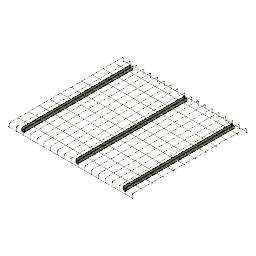
_Wire Rack.2c1b638f-f074-42f4-967c-a75b4d30ed14 (Autodesk Fusion 360 design; units mm, degrees)
Autodesk Fusion 360 part; units mm, degrees
note: some values were not read from the file. Set by a fixed rule: which sketch regions a step uses.
sketch "Sketch1" plane through (0, 0, 0) normal (1, 0, 0) x (0, 1, 0)
  circle A0 centre (0, 0) radius 2.5
  dimension "d1" = 5
  constraint coincident A0.centre origin
  measures "d1" diameter of A0
extrude "Extrude1" add sketch "Sketch1" against normal blind 1162.05 makes body 1
ref_plane "WorkPlane1" through (-4.5, 0, 0) normal (1, 0, 0) x (0, 1, 0)
sketch "Sketch2" plane through (-4.5, 0, 0) normal (1, 0, 0) x (0, 1, 0)
  circle A0 centre (0, 0) radius 2.5
  line L0 (0, 0) -> (2.5, 0)
  line L1 (5, -4.5) -> (5, 26.65)
  line L2 (11.35, 33) -> (1064.1038, 33)
  line L3 (1070.4538, 26.65) -> (1070.4538, -4.5)
  arc A1 (11.35, 33) -> (5, 26.65) centre (11.35, 26.65) ccw
  arc A2 (1070.4538, 26.65) -> (1064.1038, 33) centre (1064.1038, 26.65) ccw
  line L4 (5, -4.5) -> (-3, -4.5) construction
  point P0 (5, 33)
  point P1 (1070.4538, 33)
  dimension "d8" = 37.5
  dimension "d9" = 1065.4538
  dimension "d10" = 37.5
  dimension "d11" = 6.35
  dimension "d12" = 6.35
  constraint coincident A0.centre L0.start
  constraint coincident A0 L0.end
  constraint horizontal L0
  constraint perpendicular L1 L2
  constraint perpendicular L2 L3
  constraint coincident P0 L1
  constraint coincident P0 L2
  constraint tangent L1 A1
  constraint tangent L2 A1
  constraint coincident P1 L3
  constraint coincident P1 L2
  constraint tangent L3 A2
  constraint tangent L2 A2
  constraint perpendicular L1 L4
  measures "d8" distance of L1.start P0
  measures "d9" distance of P0 P1
  measures "d10" distance of P1 L3.end
  measures "d11" radius of A1
  measures "d12" radius of A2
ref_plane "WorkPlane2" through (-4.5, 1, -4.5) normal (0, 0, 1) x (0, -1, 0)
sketch "Sketch3" plane through (0, 0, -4.5) normal (0, 0, 1) x (1, 0, 0)
  circle A0 centre (-4.5, 5) radius 2.5
  point P0 (-4.5, 5)
  dimension "d14" = 5
  constraint coincident P0 A0.centre
  measures "d14" diameter of A0
sweep "Sweep1" add profiles "Sketch3" path "Sketch2" along L3 A2 L2 A1 L1 section 1 separate body makes body 2
ref_plane "WorkPlane3" through (-581.025, 0, 0) normal (1, 0, 0) x (0, 1, 0)
mirror "Mirror1" about plane through (-581.025, 0, 0) normal (1, 0, 0) of bodies 2 makes body 3
ref_plane "WorkPlane4" through (-2, 105.0137, 33) normal (1, 0, 0) x (0, 0, 1)
ref_plane "WorkPlane5" through (-1155.05, 336.6348, 33) normal (1, 0, 0) x (0, 0, -1)
pattern_linear "R-Pattern1" count 19 spacing 64.0583 along (1, 0, 0) of bodies 3 makes body 4 at (-1095.6567, 713.1859, 31.75) makes body 5 at (-1031.5984, 713.1859, 31.75) makes body 6 at (-967.5401, 713.1859, 31.75) makes body 7 at (-903.4817, 713.1859, 31.75) makes body 8 at (-839.4234, 713.1859, 31.75) makes body 9 at (-775.3651, 713.1859, 31.75) makes body 10 at (-711.3067, 713.1859, 31.75) makes body 11 at (-647.2484, 713.1859, 31.75) makes body 12 at (-583.1901, 713.1859, 31.75) makes body 13 at (-519.1317, 713.1859, 31.75) makes body 14 at (-455.0734, 713.1859, 31.75) makes body 15 at (-391.0151, 713.1859, 31.75) makes body 16 at (-326.9567, 713.1859, 31.75) makes body 17 at (-262.8984, 713.1859, 31.75) makes body 18 at (-198.8401, 713.1859, 31.75) makes body 19 at (-134.7817, 713.1859, 31.75) makes body 20 at (-70.7234, 713.1859, 31.75) makes body 21 at (-6.6651, 713.1859, 31.75)
delete_body "RemoveBody1" bodies 2
ref_plane "WorkPlane6" through (-260.7333, 1072.9538, 13.6481) normal (0, 1, 0) x (1, 0, 0)
ref_plane "WorkPlane7" through (-260.7333, 2.5, 19.5712) normal (0, -1, 0) x (1, 0, 0)
ref_plane "WorkPlane8" through (-260.7333, 537.7269, 13.6481) normal (0, 1, 0) x (1, 0, 0)
mirror "Mirror2" about plane through (-260.7333, 537.7269, 13.6481) normal (0, 1, 0) of bodies 1 makes body 22
combine "Combine1" operation add target body 1 tool bodies 13 12 3 5 4 11 10 9 6 7 8 14 15 16 17 18 19 20 21 22
ref_plane "WorkPlane9" through (0, 1075.4538, 0) normal (1, 0, 0) x (0, -1, 0)
ref_plane "WorkPlane10" through (-581.025, 1024.9259, 35.5) normal (0, 0, 1) x (1, 0, 0)
ref_plane "WorkPlane11" through (-1157.55, 1067.9538, 3.7896) normal (0, -1, 0) x (-1, 0, 0)
ref_plane "WorkPlane12" through (-1093.4917, 7.5, 6.3783) normal (0, 1, 0) x (-1, 0, 0)
ref_plane "WorkPlane13" through (-1162.05, 1075.4538, 0) normal (-1, 0, 0) x (0, 1, 0)
sketch "Sketch4" plane through (-1162.05, 0, 0) normal (-1, 0, 0) x (0, -1, 0)
  circle A0 centre (-1075.4538, 0) radius 2.5
  line L0 (-1064.1038, 30.5) -> (-1064.1038, 35.5)
  line L1 (-11.35, 30.5) -> (-11.35, 35.5)
  line L2 (-1075.4538, 0) -> (-986.5538, 0)
  line L3 (-1064.1038, 30.5) -> (-11.35, 30.5)
  line L4 (-986.5538, 0) -> (-986.5538, 30.5)
  circle A1 centre (-986.5538, 28) radius 2.5
  line L5 (-537.7269, 30.5) -> (-537.7269, 71.3559) construction
  circle A2 centre (-88.9, 28) radius 2.5
  dimension "d38" = 88.9
  dimension "d39" = 5
  constraint coincident A0.centre L2.start
  constraint horizontal L2
  constraint coincident L0.start L3.start
  constraint coincident L1.start L3.end
  constraint coincident L3 L4.end
  constraint perpendicular L3 L4
  constraint coincident L4.end A1
  constraint midpoint L3 L5.start
  constraint perpendicular L3 L5
  constraint symmetric A1 L5 A2
  measures "d38" distance of A0.centre L2.end
  measures "d39" diameter of A1
extrude "Extrude2" add sketch "Sketch4" against normal blind 1162.05 separate body contours L4 A1 | L4 A1 makes body 23
pattern_linear "R-Pattern2" count 10 spacing 99.7393 along (0, -1, 0) of bodies 23 makes body 24 at (-387.35, 889.2293, 28.647) makes body 25 at (-387.35, 789.4899, 28.647) makes body 26 at (-387.35, 689.7506, 28.647) makes body 27 at (-387.35, 590.0113, 28.647) makes body 28 at (-387.35, 488.5042, 30.4148) makes body 29 at (-387.35, 388.7648, 30.4148) makes body 30 at (-387.35, 289.0255, 30.4148) makes body 31 at (-387.35, 189.8891, 25.8349) makes body 32 at (-387.35, 89.5468, 30.4148)
combine "Combine2" operation add target body 1 tool bodies 30 29 26 25 23 27 24 28 32 31
ref_plane "WorkPlane14" through (-1093.4917, 30.175, 6.3783) normal (0, 1, 0) x (-1, 0, 0)
sketch "Sketch5" plane through (0, 30.175, 0) normal (0, 1, 0) x (1, 0, 0)
  circle A0 centre (-581.025, -33) radius 2.5
  circle A1 centre (-581.025, -33) radius 2.5
  circle A2 centre (-516.9667, -33) radius 2.5
  circle A3 centre (-516.9667, -33) radius 2.5
  line L0 (0, -30.5) -> (0, -25.5)
  line L1 (-1162.05, -25.5) -> (-1162.05, -30.5)
  line L2 (-516.9667, -33) -> (-516.9667, -30.5)
  line L3 (-536.2958, -30.5) -> (-536.2958, -0.1)
  line L4 (-561.6958, -30.5) -> (-561.6958, -0.1)
  line L5 (-516.9667, -30.5) -> (-536.2958, -30.5) construction
  line L6 (-561.6958, -30.5) -> (-581.025, -30.5) construction
  arc A4 (-536.2958, -0.1) -> (-561.6958, -0.1) centre (-548.9958, -0.1) ccw
  line L7 (-538.2958, -30.5) -> (-538.2958, -0.1)
  arc A5 (-538.2958, -0.1) -> (-559.6958, -0.1) centre (-548.9958, -0.1) ccw
  line L8 (-559.6958, -30.5) -> (-559.6958, -0.1)
  line L9 (-536.2958, -30.5) -> (-538.2958, -30.5)
  line L10 (-561.6958, -30.5) -> (-559.6958, -30.5)
  line L11 (0, -30.5) -> (0, -25.5)
  line L12 (-1162.05, -25.5) -> (-1162.05, -30.5)
  line L13 (-559.6958, -30.5) -> (-559.6958, -25.5)
  line L14 (-561.6958, 58.4839) -> (-536.2958, 58.4839)
  line L15 (-561.6958, -25.5) -> (-559.6958, -25.5)
  line L16 (-538.2958, -25.5) -> (-536.2958, -25.5)
  dimension "d47" = 25.4
  dimension "d49" = 25.4
  dimension "d50" = -2
  dimension "d60" = 5
  dimension "d61" = 30.4
  constraint coincident A2.centre A3.centre
  constraint coincident A3 L2.end
  constraint vertical L2
  constraint coincident A0 L6.end
  constraint tangent A0 L6
  constraint tangent L3 A4
  constraint tangent L4 A4
  constraint collinear L5 L6
  constraint perpendicular L10 L13
  constraint coincident L4 L14.start
  constraint coincident L3 L14.end
  constraint perpendicular L3 L14
  constraint coincident L4 L15.start
  constraint perpendicular L8 L15
  constraint coincident L7 L16.start
  constraint coincident L3 L16.end
  constraint perpendicular L3 L16
  measures "d47" distance of L3.start L4.start
  measures "d49" diameter of A4
  measures "d60" distance of L8.start L13.end
  measures "d61" distance of L4.start L4.end
ref_plane "WorkPlane15" through (-68.5583, 1067.9538, 15.8554) normal (0, -1, 0) x (-1, 0, 0)
ref_plane "WorkPlane16" through (-68.5583, 1045.2788, 15.8554) normal (0, -1, 0) x (-1, 0, 0)
extrude "Extrude3" add sketch "Sketch5" along normal blind 1015.104 separate body contours L3 L4 A4 L7 A5 L8 L15 L16 makes body 33
ref_plane "WorkPlane17" through (-548.9958, 985.3992, -12.6) normal (0, 0, -1) x (1, 0, 0)
sketch "Sketch6" plane through (0, 0, -12.6) normal (0, 0, -1) x (-1, 0, 0)
  line L0 (561.6958, 30.175) -> (536.2958, 30.175)
  line L1 (561.6958, 30.175) -> (561.6958, 1045.279)
  line L2 (561.6958, 1045.279) -> (536.2958, 1045.279)
  line L3 (536.2958, 1045.279) -> (536.2958, 30.175)
  line L4 (548.9958, 1045.279) -> (548.9958, 1033.279)
  circle A0 centre (548.9958, 1033.279) radius 3.5
  line L5 (536.2958, 537.727) -> (561.6958, 537.727) construction
  line L6 (536.2958, 537.727) -> (561.6958, 537.727) construction
  circle A1 centre (548.9958, 42.175) radius 3.5
  dimension "d56" = 12
  dimension "d57" = 7
  constraint midpoint L2 L4.start
  constraint perpendicular L2 L4
  constraint coincident L4.end A0.centre
  constraint midpoint L3 L5.start
  constraint midpoint L1 L5.end
  constraint symmetric A0 L5 A1
  constraint symmetric L6.start L5 L5.start
  constraint symmetric L6.end L5 L5.end
  measures "d56" distance of L4.start L4.end
  measures "d57" diameter of A0
extrude "Extrude4" cut sketch "Sketch6" along normal mid plane 160 contours A0 | A1 bodies 33
pattern_linear "R-Pattern3" count 2 spacing 444.5 along (1, 0, 0) of bodies 33 makes body 34
pattern_linear "R-Pattern4" count 2 spacing 508 along (-1, 0, 0) of bodies 33 makes body 35
equation "d47 = 1\""
equation "d49 = 1\""
equation "d68 = -20\""
